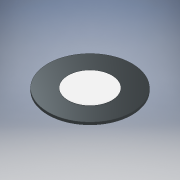
# Autodesk Inventor part: lid
Saved by Autodesk Inventor 2020 (Build 240168000, 168)
## iProperties
Created: 2024-12-06
Part Number: lid
Material: Полиэтилен, низкая плотность
Document SubType Name: Modeling
Designer: Ivan
Density: 0.894 g/cm^3
Appearance: Чугун серый
Author: Ivan
Autodesk Inventor part; units mm, degrees
ref_plane "YZ Plane" through (0, 0, 0) normal (1, 0, 0) x (0, 1, 0)
ref_plane "XZ Plane" through (0, 0, 0) normal (0, 1, 0) x (-1, 0, 0)
ref_plane "XY Plane" through (0, 0, 0) normal (0, 0, 1) x (1, 0, 0)
sketch "Эскиз6" plane through (0, 0, 0) normal (0, 1, 0) x (-1, 0, 0)
  circle A0 centre (0, 0) radius 27
  circle A1 centre (0, 0) radius 29.1
  circle A2 centre (0, 0) radius 52
  circle A3 centre (0, 0) radius 31.6
  dimension "d16" = 54
  dimension "d17" = 58.2
  dimension "d18" = 104
  dimension "d23" = 63.2
  constraints: 6 coincident, 4 centre point
  measures "d16" diameter of A0
  measures "d17" diameter of A1
  measures "d18" diameter of A2
  measures "d23" diameter of A3
extrude "Выдавливание4" add sketch "Эскиз6" along normal blind 4.7 contours A0 | A1 | A2 | A3
extrude "Выдавливание5" cut sketch "Эскиз6" along normal blind 2.5 contours A1
extrude "Выдавливание6" cut sketch "Эскиз6" along normal blind 1.7 contours A2
chamfer "Фаска1" distance 1.2 angle 45 1 edges at (31.6, 0, 0)
sketch "Эскиз7" plane through (0, 4.7, 0) normal (0, 1, 0) x (1, 0, 0)
  circle A0 centre (0, 0) radius 27 projected
extrude "Выдавливание7" add sketch "Эскиз7" along normal blind 0.05 and the other way blind 0.1 separate body
